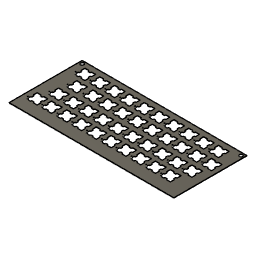
Metal_dome_array_layer_0.4mm (Autodesk Fusion 360 design; units mm, degrees)
Autodesk Fusion 360 part; units mm, degrees
(part 1 of 4)
sketch "스케치1" plane through (0, 0, 0) normal (0, 0, 1) x (1, 0, 0)
  line L0 (0, 69) -> (155.5, 69)
  line L1 (155.5, 69) -> (155.5, 0)
  line L2 (155.5, 0) -> (0, 0)
  line L3 (0, 0) -> (0, 69)
  line L4 (12.673, 10.08) -> (26.673, 10.08) construction
  line L5 (26.673, 10.08) -> (40.673, 10.08) construction
  line L6 (40.673, 10.08) -> (54.673, 10.08) construction
  line L7 (54.673, 10.08) -> (68.673, 10.08) construction
  line L8 (68.673, 10.08) -> (82.673, 10.08) construction
  line L9 (82.673, 10.08) -> (96.673, 10.08) construction
  line L10 (96.673, 10.08) -> (110.673, 10.08) construction
  line L11 (110.673, 10.08) -> (124.673, 10.08) construction
  line L12 (124.673, 10.08) -> (138.673, 10.08) construction
  circle A0 centre (12.673, 10.08) radius 5.05
  circle A1 centre (26.673, 10.08) radius 5.05
  circle A2 centre (40.673, 10.08) radius 5.05
  circle A3 centre (54.673, 10.08) radius 5.05
  circle A4 centre (68.673, 10.08) radius 5.05
  circle A5 centre (82.673, 10.08) radius 5.05
  circle A6 centre (96.673, 10.08) radius 5.05
  circle A7 centre (110.673, 10.08) radius 5.05
  circle A8 centre (124.673, 10.08) radius 5.05
  circle A9 centre (138.673, 10.08) radius 5.05
  line L13 (19.024, 24.05) -> (34.274, 24.05) construction
  line L14 (34.274, 24.05) -> (48.244, 24.05) construction
  line L15 (48.244, 24.05) -> (62.214, 24.05) construction
  line L16 (62.214, 24.05) -> (76.184, 24.05) construction
  line L17 (76.184, 24.05) -> (90.154, 24.05) construction
  line L18 (90.154, 24.05) -> (104.124, 24.05) construction
  line L19 (104.124, 24.05) -> (118.094, 24.05) construction
  line L20 (118.094, 24.05) -> (132.064, 24.05) construction
  line L21 (132.064, 24.05) -> (146.034, 24.05) construction
  circle A10 centre (19.024, 24.05) radius 5.05
  circle A11 centre (34.274, 24.05) radius 5.05
  circle A12 centre (48.244, 24.05) radius 5.05
  circle A13 centre (62.214, 24.05) radius 5.05
  circle A14 centre (76.184, 24.05) radius 5.05
  circle A15 centre (90.154, 24.05) radius 5.05
  circle A16 centre (104.124, 24.05) radius 5.05
  circle A17 centre (118.094, 24.05) radius 5.05
  circle A18 centre (132.064, 24.05) radius 5.05
  circle A19 centre (146.034, 24.05) radius 5.05
  line L22 (16.483, 38.655) -> (30.453, 38.655) construction
  line L23 (30.453, 38.655) -> (44.423, 38.655) construction
  line L24 (44.423, 38.655) -> (58.393, 38.655) construction
  line L25 (58.393, 38.655) -> (72.363, 38.655) construction
  circle A20 centre (16.483, 38.655) radius 5.05
  circle A21 centre (30.453, 38.655) radius 5.05
  circle A22 centre (44.423, 38.655) radius 5.05
  circle A23 centre (58.393, 38.655) radius 5.05
  circle A24 centre (72.363, 38.655) radius 5.05
  circle A25 centre (86.333, 38.655) radius 5.05
  circle A26 centre (100.303, 38.655) radius 5.05
  circle A27 centre (114.273, 38.655) radius 5.05
  circle A28 centre (128.243, 38.655) radius 5.05
  circle A29 centre (142.213, 38.655) radius 5.05
  line L26 (72.363, 38.655) -> (86.333, 38.655) construction
  line L27 (86.333, 38.655) -> (100.303, 38.655) construction
  line L28 (100.303, 38.655) -> (114.273, 38.655) construction
  line L29 (114.273, 38.655) -> (128.243, 38.655) construction
  line L30 (128.243, 38.655) -> (142.213, 38.655) construction
  line L31 (10.13, 52.625) -> (23.78, 52.625) construction
  line L32 (23.78, 52.625) -> (38.07, 52.625) construction
  line L33 (38.07, 52.625) -> (52.04, 52.625) construction
  line L34 (52.04, 52.625) -> (66.01, 52.625) construction
  line L35 (66.01, 52.625) -> (79.98, 52.625) construction
  line L36 (79.98, 52.625) -> (93.95, 52.625) construction
  line L37 (93.95, 52.625) -> (107.92, 52.625) construction
  line L38 (107.92, 52.625) -> (121.89, 52.625) construction
  line L39 (121.89, 52.625) -> (135.86, 52.625) construction
  circle A30 centre (10.13, 52.625) radius 5.05
  circle A31 centre (23.78, 52.625) radius 5.05
  circle A32 centre (38.07, 52.625) radius 5.05
  circle A33 centre (52.04, 52.625) radius 5.05
  circle A34 centre (79.98, 52.625) radius 5.05
  circle A35 centre (93.95, 52.625) radius 5.05
  circle A36 centre (107.92, 52.625) radius 5.05
  circle A37 centre (121.89, 52.625) radius 5.05
  circle A38 centre (135.86, 52.625) radius 5.05
  circle A39 centre (66.01, 52.625) radius 5.05
  circle A40 centre (2.8, 2.8) radius 1.55
  circle A41 centre (152.7, 2.8) radius 1.55
  circle A42 centre (3.81, 65.25) radius 0.95
  circle A43 centre (151.69, 65.25) radius 0.95
  line L40 (0.4, 68.6) -> (155.1, 68.6)
  line L41 (155.1, 68.6) -> (155.1, 0.4)
  line L42 (155.1, 0.4) -> (0.4, 0.4)
  line L43 (0.4, 0.4) -> (0.4, 68.6)
  dimension "d1" = 155.5
  dimension "d2" = 69
  dimension "d3" = 14
  dimension "d4" = 12.673
  dimension "d5" = 10.08
  dimension "d6" = 10.1
  dimension "d8" = 15.25
  dimension "d9" = 13.97
  dimension "d10" = 19.024
  dimension "d11" = 13.97
  dimension "d12" = 13.97
  dimension "d13" = 14.605
  dimension "d14" = 16.483
  dimension "d15" = 13.65
  dimension "d16" = 14.29
  dimension "d17" = 13.97
  dimension "d18" = 10.13
  dimension "d19" = 13.97
  dimension "d20" = 3.1
  dimension "d21" = 2.8
  dimension "d22" = 2.8
  dimension "d23" = 2.8
  dimension "d24" = 2.8
  dimension "d25" = 3.81
  dimension "d26" = 65.25
  dimension "d27" = 1.9
  dimension "d28" = 3.81
  dimension "d29" = 65.25
  dimension "d45" = 0.4
  constraint horizontal L0
  constraint vertical L1
  constraint horizontal L2
  constraint vertical L3
  constraint coincident L2.end L3.start
  constraint horizontal L4
  constraint parallel L4 L5
  constraint parallel L5 L6
  constraint parallel L6 L7
  constraint parallel L6 L8
  constraint parallel L8 L9
  constraint parallel L8 L10
  constraint parallel L10 L11
  constraint parallel L10 L12
  constraint equal L4 L5
  constraint equal L4 L6
  constraint equal L4 L7
  constraint equal L4 L8
  constraint equal L4 L9
  constraint equal L4 L10
  constraint equal L4 L11
  constraint equal L4 L12
  constraint coincident L4.start A0.centre
  constraint coincident L4.end L5.start
  constraint coincident L5.end L6.start
  constraint coincident L6.end L7.start
  constraint coincident L7.end L8.start
  constraint coincident L8.end L9.start
  constraint coincident L9.end L10.start
  constraint coincident L10.end L11.start
  constraint coincident L11.end L12.start
  constraint coincident L12.end A9.centre
  constraint equal A0 A1
  constraint equal A0 A2
  constraint equal A0 A3
  constraint equal A0 A4
  constraint equal A0 A5
  constraint equal A0 A6
  constraint equal A0 A7
  constraint equal A0 A8
  constraint equal A0 A9
  constraint parallel L0 L13
  constraint parallel L0 L14
  constraint parallel L0 L15
  constraint parallel L15 L16
  constraint parallel L16 L17
  constraint parallel L16 L18
  constraint parallel L18 L19
  constraint parallel L18 L20
  constraint parallel L18 L21
  constraint equal L15 L16
  constraint equal L15 L17
  constraint equal L15 L18
  constraint equal L15 L19
  constraint equal L15 L20
  constraint equal L15 L21
  constraint equal L14 L15
  constraint coincident L21.end A19.centre
  constraint coincident L20.end L21.start
  constraint coincident L19.end L20.start
  constraint coincident L18.end L19.start
  constraint coincident L17.end L18.start
  constraint coincident L16.end L17.start
  constraint coincident L15.end L16.start
  constraint coincident L14.end L15.start
  constraint coincident L13.end L14.start
  constraint coincident L13.start A10.centre
  constraint equal A0 A10
  constraint equal A0 A11
  constraint equal A0 A12
  constraint equal A0 A13
  constraint equal A0 A14
  constraint equal A0 A15
  constraint equal A0 A16
  constraint equal A0 A17
  constraint equal A0 A18
  constraint equal A0 A19
  constraint horizontal L22
  constraint parallel L22 L23
  constraint parallel L23 L24
  constraint parallel L24 L25
  constraint equal L22 L23
  constraint equal L22 L24
  constraint equal L22 L25
  constraint coincident L22.start A20.centre
  constraint coincident L22.end L23.start
  constraint coincident L23.end L24.start
  constraint coincident L24.end L25.start
  constraint coincident L25.end A24.centre
  constraint parallel L25 L26
  constraint parallel L25 L27
  constraint parallel L25 L28
  constraint parallel L25 L29
  constraint parallel L25 L30
  constraint equal L22 L26
  constraint equal L22 L27
  constraint equal L22 L28
  constraint equal L22 L29
  constraint coincident A25.centre L26.end
  constraint coincident A26.centre L27.end
  constraint coincident A27.centre L28.end
  constraint coincident A28.centre L29.end
  constraint coincident A29.centre L30.end
  constraint equal L22 L30
  constraint equal A0 A20
  constraint equal A0 A21
  constraint equal A0 A22
  constraint equal A0 A23
  constraint equal A0 A24
  constraint equal A0 A25
  constraint equal A0 A26
  constraint equal A0 A27
  constraint equal A0 A28
  constraint equal A0 A29
  constraint horizontal L31
  constraint parallel L31 L32
  constraint parallel L32 L33
  constraint parallel L33 L34
  constraint parallel L33 L35
  constraint parallel L35 L36
  constraint parallel L36 L37
  constraint parallel L37 L38
  constraint parallel L38 L39
  constraint equal L33 L34
  constraint equal L33 L35
  constraint equal L33 L36
  constraint equal L33 L37
  constraint equal L33 L38
  constraint equal L33 L39
  constraint coincident L31.start A30.centre
  constraint coincident L31.end L32.start
  constraint coincident L32.end L33.start
  constraint coincident L33.end L34.start
  constraint coincident L34.end L35.start
  constraint coincident L35.end L36.start
  constraint coincident L36.end L37.start
  constraint coincident L37.end L38.start
  constraint coincident L38.end L39.start
  constraint coincident L39.end A38.centre
  constraint equal A0 A30
  constraint equal A0 A31
  constraint equal A0 A32
  constraint equal A0 A33
  constraint equal A0 A39
  constraint equal A0 A34
  constraint equal A0 A35
  constraint equal A0 A36
  constraint equal A0 A37
  constraint equal A0 A38
  constraint equal A40 A41
  constraint equal A42 A43
  measures "d1" distance of L1.end L2.end
  measures "d2" distance of L0.start L2.end
  measures "d3" distance of L4.start L4.end
  measures "d4" distance of L3 L4.start
  measures "d5" distance of L2 L4.start
  measures "d6" diameter of A0
  measures "d8" distance of L13.start L13.end
  measures "d9" distance of L13.end L14.end
  measures "d10" distance of L3 L13.start
  measures "d11" distance of L4 L13.start
  measures "d12" distance of L22.start L22.end
  measures "d13" distance of L13 L22.start
  measures "d14" distance of L3 L22.start
  measures "d15" distance of L31.start L31.end
  measures "d16" distance of L31.end L32.end
  measures "d17" distance of L32.end L33.end
  measures "d18" distance of L3 L31.start
  measures "d19" distance of L22 L31.start
  measures "d20" diameter of A40
  measures "d21" distance of L2 A40.centre
  measures "d22" distance of L3 A40.centre
  measures "d23" distance of L2 A41.centre
  measures "d24" distance of L1 A41.centre
  measures "d25" distance of L3 A42.centre
  measures "d26" distance of L2 A42.centre
  measures "d27" diameter of A42
  measures "d28" distance of L1 A43.centre
  measures "d29" distance of L2 A43.centre
sketch "스케치2" plane through (0, 0, 0) normal (0, 0, 1) x (1, 0, 0)
  line L0 (5.08, 57.675) -> (15.18, 57.675)
  line L1 (15.18, 57.675) -> (15.18, 47.575)
  line L2 (15.18, 47.575) -> (5.08, 47.575)
  line L3 (5.08, 47.575) -> (5.08, 57.675)
  line L4 (18.73, 57.675) -> (28.83, 57.675)
  line L5 (28.83, 57.675) -> (28.83, 47.575)
  line L6 (28.83, 47.575) -> (18.73, 47.575)
  line L7 (18.73, 47.575) -> (18.73, 57.675)
  line L8 (33.02, 57.675) -> (43.12, 57.675)
  line L9 (43.12, 57.675) -> (43.12, 47.575)
  line L10 (43.12, 47.575) -> (33.02, 47.575)
  line L11 (33.02, 47.575) -> (33.02, 57.675)
  line L12 (46.99, 57.675) -> (57.09, 57.675)
  line L13 (57.09, 57.675) -> (57.09, 47.575)
  line L14 (57.09, 47.575) -> (46.99, 47.575)
  line L15 (46.99, 47.575) -> (46.99, 57.675)
  line L16 (60.96, 57.675) -> (71.06, 57.675)
  line L17 (71.06, 57.675) -> (71.06, 47.575)
  line L18 (71.06, 47.575) -> (60.96, 47.575)
  line L19 (60.96, 47.575) -> (60.96, 57.675)
  line L20 (74.93, 57.675) -> (85.03, 57.675)
  line L21 (85.03, 57.675) -> (85.03, 47.575)
  line L22 (85.03, 47.575) -> (74.93, 47.575)
  line L23 (74.93, 47.575) -> (74.93, 57.675)
  line L24 (88.9, 57.675) -> (99, 57.675)
  line L25 (99, 57.675) -> (99, 47.575)
  line L26 (99, 47.575) -> (88.9, 47.575)
  line L27 (88.9, 47.575) -> (88.9, 57.675)
  line L28 (102.87, 57.675) -> (112.97, 57.675)
  line L29 (112.97, 57.675) -> (112.97, 47.575)
  line L30 (112.97, 47.575) -> (102.87, 47.575)
  line L31 (102.87, 47.575) -> (102.87, 57.675)
  line L32 (116.84, 57.675) -> (126.94, 57.675)
  line L33 (126.94, 57.675) -> (126.94, 47.575)
  line L34 (126.94, 47.575) -> (116.84, 47.575)
  line L35 (116.84, 47.575) -> (116.84, 57.675)
  line L36 (130.81, 57.675) -> (140.91, 57.675)
  line L37 (140.91, 57.675) -> (140.91, 47.575)
  line L38 (140.91, 47.575) -> (130.81, 47.575)
  line L39 (130.81, 47.575) -> (130.81, 57.675)
  line L40 (11.433, 43.705) -> (21.533, 43.705)
  line L41 (21.533, 43.705) -> (21.533, 33.605)
  line L42 (21.533, 33.605) -> (11.433, 33.605)
  line L43 (11.433, 33.605) -> (11.433, 43.705)
  line L44 (25.403, 43.705) -> (35.503, 43.705)
  line L45 (35.503, 43.705) -> (35.503, 33.605)
  line L46 (35.503, 33.605) -> (25.403, 33.605)
  line L47 (25.403, 33.605) -> (25.403, 43.705)
  line L48 (39.373, 43.705) -> (49.473, 43.705)
  line L49 (49.473, 43.705) -> (49.473, 33.605)
  line L50 (49.473, 33.605) -> (39.373, 33.605)
  line L51 (39.373, 33.605) -> (39.373, 43.705)
  line L52 (53.343, 43.705) -> (63.443, 43.705)
  line L53 (63.443, 43.705) -> (63.443, 33.605)
  line L54 (63.443, 33.605) -> (53.343, 33.605)
  line L55 (53.343, 33.605) -> (53.343, 43.705)
  line L56 (67.313, 43.705) -> (77.413, 43.705)
  line L57 (77.413, 43.705) -> (77.413, 33.605)
  line L58 (77.413, 33.605) -> (67.313, 33.605)
  line L59 (67.313, 33.605) -> (67.313, 43.705)
  line L60 (81.283, 43.705) -> (91.383, 43.705)
  line L61 (91.383, 43.705) -> (91.383, 33.605)
  line L62 (91.383, 33.605) -> (81.283, 33.605)
  line L63 (81.283, 33.605) -> (81.283, 43.705)
  line L64 (95.253, 43.705) -> (105.353, 43.705)
  line L65 (105.353, 43.705) -> (105.353, 33.605)
  line L66 (105.353, 33.605) -> (95.253, 33.605)
  line L67 (95.253, 33.605) -> (95.253, 43.705)
  line L68 (109.223, 43.705) -> (119.323, 43.705)
  line L69 (119.323, 43.705) -> (119.323, 33.605)
  line L70 (119.323, 33.605) -> (109.223, 33.605)
  line L71 (109.223, 33.605) -> (109.223, 43.705)
  line L72 (123.193, 43.705) -> (133.293, 43.705)
  line L73 (133.293, 43.705) -> (133.293, 33.605)
  line L74 (133.293, 33.605) -> (123.193, 33.605)
  line L75 (123.193, 33.605) -> (123.193, 43.705)
  line L76 (137.163, 43.705) -> (147.263, 43.705)
  line L77 (147.263, 43.705) -> (147.263, 33.605)
  line L78 (147.263, 33.605) -> (137.163, 33.605)
  line L79 (137.163, 33.605) -> (137.163, 43.705)
  line L80 (140.984, 29.1) -> (151.084, 29.1)
  line L81 (151.084, 29.1) -> (151.084, 19)
  line L82 (151.084, 19) -> (140.984, 19)
  line L83 (140.984, 19) -> (140.984, 29.1)
  line L84 (127.014, 29.1) -> (137.114, 29.1)
  line L85 (137.114, 29.1) -> (137.114, 19)
  line L86 (137.114, 19) -> (127.014, 19)
  line L87 (127.014, 19) -> (127.014, 29.1)
  line L88 (113.044, 29.1) -> (123.144, 29.1)
  line L89 (123.144, 29.1) -> (123.144, 19)
  line L90 (123.144, 19) -> (113.044, 19)
  line L91 (113.044, 19) -> (113.044, 29.1)
  line L92 (99.074, 29.1) -> (109.174, 29.1)
  line L93 (109.174, 29.1) -> (109.174, 19)
  line L94 (109.174, 19) -> (99.074, 19)
  line L95 (99.074, 19) -> (99.074, 29.1)
  line L96 (85.104, 29.1) -> (95.204, 29.1)
  line L97 (95.204, 29.1) -> (95.204, 19)
  line L98 (95.204, 19) -> (85.104, 19)
  line L99 (85.104, 19) -> (85.104, 29.1)
  line L100 (71.134, 29.1) -> (81.234, 29.1)
  line L101 (81.234, 29.1) -> (81.234, 19)
  line L102 (81.234, 19) -> (71.134, 19)
  line L103 (71.134, 19) -> (71.134, 29.1)
  line L104 (57.164, 29.1) -> (67.264, 29.1)
  line L105 (67.264, 29.1) -> (67.264, 19)
  line L106 (67.264, 19) -> (57.164, 19)
  line L107 (57.164, 19) -> (57.164, 29.1)
  line L108 (43.194, 29.1) -> (53.294, 29.1)
  line L109 (53.294, 29.1) -> (53.294, 19)
  line L110 (53.294, 19) -> (43.194, 19)
  line L111 (43.194, 19) -> (43.194, 29.1)
  line L112 (29.224, 29.1) -> (39.324, 29.1)
  line L113 (39.324, 29.1) -> (39.324, 19)
  line L114 (39.324, 19) -> (29.224, 19)
  line L115 (29.224, 19) -> (29.224, 29.1)
  line L116 (13.974, 29.1) -> (24.074, 29.1)
  line L117 (24.074, 29.1) -> (24.074, 19)
  line L118 (24.074, 19) -> (13.974, 19)
  line L119 (13.974, 19) -> (13.974, 29.1)
  line L120 (7.623, 15.13) -> (17.723, 15.13)
  line L121 (17.723, 15.13) -> (17.723, 5.03)
  line L122 (17.723, 5.03) -> (7.623, 5.03)
  line L123 (7.623, 5.03) -> (7.623, 15.13)
  line L124 (21.623, 15.13) -> (31.723, 15.13)
  line L125 (31.723, 15.13) -> (31.723, 5.03)
  line L126 (31.723, 5.03) -> (21.623, 5.03)
  line L127 (21.623, 5.03) -> (21.623, 15.13)
  line L128 (35.623, 15.13) -> (45.723, 15.13)
  line L129 (45.723, 15.13) -> (45.723, 5.03)
  line L130 (45.723, 5.03) -> (35.623, 5.03)
  line L131 (35.623, 5.03) -> (35.623, 15.13)
  line L132 (49.623, 15.13) -> (59.723, 15.13)
  line L133 (59.723, 15.13) -> (59.723, 5.03)
  line L134 (59.723, 5.03) -> (49.623, 5.03)
  line L135 (49.623, 5.03) -> (49.623, 15.13)
  line L136 (63.623, 15.13) -> (73.723, 15.13)
  line L137 (73.723, 15.13) -> (73.723, 5.03)
  line L138 (73.723, 5.03) -> (63.623, 5.03)
  line L139 (63.623, 5.03) -> (63.623, 15.13)
  line L140 (77.623, 15.13) -> (87.723, 15.13)
  line L141 (87.723, 15.13) -> (87.723, 5.03)
  line L142 (87.723, 5.03) -> (77.623, 5.03)
  line L143 (77.623, 5.03) -> (77.623, 15.13)
  line L144 (91.623, 15.13) -> (101.723, 15.13)
  line L145 (101.723, 15.13) -> (101.723, 5.03)
  line L146 (101.723, 5.03) -> (91.623, 5.03)
  line L147 (91.623, 5.03) -> (91.623, 15.13)
  line L148 (105.623, 15.13) -> (115.723, 15.13)
  line L149 (115.723, 15.13) -> (115.723, 5.03)
  line L150 (115.723, 5.03) -> (105.623, 5.03)
  line L151 (105.623, 5.03) -> (105.623, 15.13)
  line L152 (119.623, 15.13) -> (129.723, 15.13)
  line L153 (129.723, 15.13) -> (129.723, 5.03)
  line L154 (129.723, 5.03) -> (119.623, 5.03)
  line L155 (119.623, 5.03) -> (119.623, 15.13)
  line L156 (133.623, 15.13) -> (143.723, 15.13)
  line L157 (143.723, 15.13) -> (143.723, 5.03)
  line L158 (143.723, 5.03) -> (133.623, 5.03)
  line L159 (133.623, 5.03) -> (133.623, 15.13)
  circle A0 centre (10.13, 52.625) radius 5.05
  circle A1 centre (23.78, 52.625) radius 5.05
  circle A2 centre (38.07, 52.625) radius 5.05
  circle A3 centre (52.04, 52.625) radius 5.05
  circle A4 centre (66.01, 52.625) radius 5.05
  circle A5 centre (79.98, 52.625) radius 5.05
  circle A6 centre (93.95, 52.625) radius 5.05
  circle A7 centre (107.92, 52.625) radius 5.05
  circle A8 centre (121.89, 52.625) radius 5.05
  circle A9 centre (135.86, 52.625) radius 5.05
  circle A10 centre (16.483, 38.655) radius 5.05
  circle A11 centre (30.453, 38.655) radius 5.05
  circle A12 centre (44.423, 38.655) radius 5.05
  circle A13 centre (58.393, 38.655) radius 5.05
  circle A14 centre (72.363, 38.655) radius 5.05
  circle A15 centre (86.333, 38.655) radius 5.05
  circle A16 centre (100.303, 38.655) radius 5.05
  circle A17 centre (114.273, 38.655) radius 5.05
  circle A18 centre (128.243, 38.655) radius 5.05
  circle A19 centre (142.213, 38.655) radius 5.05
  circle A20 centre (19.024, 24.05) radius 5.05
  circle A21 centre (34.274, 24.05) radius 5.05
  circle A22 centre (48.244, 24.05) radius 5.05
  circle A23 centre (76.184, 24.05) radius 5.05
  circle A24 centre (62.214, 24.05) radius 5.05
  circle A25 centre (90.154, 24.05) radius 5.05
  circle A26 centre (104.124, 24.05) radius 5.05
  circle A27 centre (118.094, 24.05) radius 5.05
  circle A28 centre (132.064, 24.05) radius 5.05
  circle A29 centre (146.034, 24.05) radius 5.05
  circle A30 centre (12.673, 10.08) radius 5.05
  circle A31 centre (26.673, 10.08) radius 5.05
  circle A32 centre (40.673, 10.08) radius 5.05
  circle A33 centre (54.673, 10.08) radius 5.05
  circle A34 centre (68.673, 10.08) radius 5.05
  circle A35 centre (82.673, 10.08) radius 5.05
  circle A36 centre (96.673, 10.08) radius 5.05
  circle A37 centre (110.673, 10.08) radius 5.05
  circle A38 centre (124.673, 10.08) radius 5.05
  circle A39 centre (138.673, 10.08) radius 5.05
  line L160 (5.08, 55.7658) -> (6.9892, 57.675)
  line L161 (6.0346, 56.7204) -> (5.08, 57.675) construction
  line L162 (137.163, 41.7958) -> (139.0722, 43.705)
  line L163 (137.163, 43.705) -> (137.3462, 43.705) construction
  line L164 (137.163, 43.705) -> (138.1176, 42.7504) construction
  line L165 (13.974, 27.1908) -> (15.8832, 29.1)
  line L166 (13.974, 29.1) -> (14.9286, 28.1454) construction
  line L167 (133.623, 13.2208) -> (135.5322, 15.13)
  line L168 (133.623, 15.13) -> (134.5776, 14.1754) construction
  circle A40 centre (5.7164, 57.0386) radius 0.45
  circle A41 centre (14.6104, 28.4636) radius 0.45
  circle A42 centre (137.7994, 43.0686) radius 0.45
  circle A43 centre (134.2594, 14.4936) radius 0.45
  line L169 (25.403, 41.7958) -> (27.3122, 43.705)
  line L170 (53.343, 41.7958) -> (55.2522, 43.705)
  line L171 (81.283, 41.7958) -> (83.1922, 43.705)
  line L172 (109.223, 41.7958) -> (111.1322, 43.705)
  line L173 (43.194, 27.1908) -> (45.1032, 29.1)
  line L174 (18.73, 55.7658) -> (20.6392, 57.675)
  line L175 (33.02, 55.7658) -> (34.9292, 57.675)
  line L176 (46.99, 55.7658) -> (48.8992, 57.675)
  line L177 (60.96, 55.7658) -> (62.8692, 57.675)
  line L178 (74.93, 55.7658) -> (76.8392, 57.675)
  line L179 (88.9, 55.7658) -> (90.8092, 57.675)
  line L180 (102.87, 55.7658) -> (104.7792, 57.675)
  line L181 (116.84, 55.7658) -> (118.7492, 57.675)
  line L182 (130.81, 55.7658) -> (132.7192, 57.675)
  line L183 (18.73, 57.675) -> (19.6846, 56.7204) construction
  line L184 (33.02, 57.675) -> (33.9746, 56.7204) construction
  line L185 (46.99, 57.675) -> (47.9446, 56.7204) construction
  line L186 (60.96, 57.675) -> (61.9146, 56.7204) construction
  line L187 (74.93, 57.675) -> (75.8846, 56.7204) construction
  line L188 (88.9, 57.675) -> (89.8546, 56.7204) construction
  line L189 (102.87, 57.675) -> (103.8246, 56.7204) construction
  line L190 (116.84, 57.675) -> (117.7946, 56.7204) construction
  line L191 (130.81, 57.675) -> (131.7646, 56.7204) construction
  circle A44 centre (19.3664, 57.0386) radius 0.45
  circle A45 centre (33.6564, 57.0386) radius 0.45
  circle A46 centre (47.6264, 57.0386) radius 0.45
  circle A47 centre (61.5964, 57.0386) radius 0.45
  circle A48 centre (75.5664, 57.0386) radius 0.45
  circle A49 centre (89.5364, 57.0386) radius 0.45
  circle A50 centre (103.5064, 57.0386) radius 0.45
  circle A51 centre (117.4764, 57.0386) radius 0.45
  circle A52 centre (131.4464, 57.0386) radius 0.45
  line L192 (11.433, 41.7958) -> (13.3422, 43.705)
  line L193 (39.373, 41.7958) -> (41.2822, 43.705)
  line L194 (67.313, 41.7958) -> (69.2222, 43.705)
  line L195 (95.253, 41.7958) -> (97.1622, 43.705)
  line L196 (123.193, 41.7958) -> (125.1022, 43.705)
  line L197 (11.433, 43.705) -> (12.3876, 42.7504) construction
  line L198 (25.403, 43.705) -> (26.3576, 42.7504) construction
  line L199 (39.373, 43.705) -> (40.3276, 42.7504) construction
  line L200 (53.343, 43.705) -> (54.2976, 42.7504) construction
  line L201 (67.313, 43.705) -> (68.2676, 42.7504) construction
  line L202 (81.283, 43.705) -> (82.2376, 42.7504) construction
  line L203 (95.253, 43.705) -> (96.2076, 42.7504) construction
  line L204 (109.223, 43.705) -> (110.1776, 42.7504) construction
  line L205 (123.193, 43.705) -> (124.1476, 42.7504) construction
  circle A53 centre (12.0694, 43.0686) radius 0.45
  circle A54 centre (26.0394, 43.0686) radius 0.45
  circle A55 centre (40.0094, 43.0686) radius 0.45
  circle A56 centre (53.9794, 43.0686) radius 0.45
  circle A57 centre (67.9494, 43.0686) radius 0.45
  circle A58 centre (81.9194, 43.0686) radius 0.45
  circle A59 centre (95.8894, 43.0686) radius 0.45
  circle A60 centre (109.8594, 43.0686) radius 0.45
  circle A61 centre (123.8294, 43.0686) radius 0.45
  line L206 (29.224, 27.1908) -> (31.1332, 29.1)
  line L207 (57.164, 27.1908) -> (59.0732, 29.1)
  line L208 (71.134, 27.1908) -> (73.0432, 29.1)
  line L209 (85.104, 27.1908) -> (87.0132, 29.1)
  line L210 (99.074, 27.1908) -> (100.9832, 29.1)
  line L211 (113.044, 27.1908) -> (114.9532, 29.1)
  line L212 (127.014, 27.1908) -> (128.9232, 29.1)
  line L213 (140.984, 27.1908) -> (142.8932, 29.1)
  line L214 (127.014, 29.1) -> (127.9686, 28.1454) construction
  line L215 (113.044, 29.1) -> (113.9986, 28.1454) construction
  line L216 (99.074, 29.1) -> (100.0286, 28.1454) construction
  line L217 (85.104, 29.1) -> (86.0586, 28.1454) construction
  line L218 (71.134, 29.1) -> (72.0886, 28.1454) construction
  line L219 (57.164, 29.1) -> (58.1186, 28.1454) construction
  line L220 (43.194, 29.1) -> (44.1486, 28.1454) construction
  line L221 (29.224, 29.1) -> (30.1786, 28.1454) construction
  line L222 (140.984, 29.1) -> (141.9386, 28.1454) construction
  circle A62 centre (29.8604, 28.4636) radius 0.45
  circle A63 centre (57.8004, 28.4636) radius 0.45
  circle A64 centre (43.8304, 28.4636) radius 0.45
  circle A65 centre (85.7404, 28.4636) radius 0.45
  circle A66 centre (71.7704, 28.4636) radius 0.45
  circle A67 centre (113.6804, 28.4636) radius 0.45
  circle A68 centre (99.7104, 28.4636) radius 0.45
  circle A69 centre (141.6204, 28.4636) radius 0.45
  circle A70 centre (127.6504, 28.4636) radius 0.45
  line L223 (119.623, 13.2208) -> (121.5322, 15.13)
  line L224 (105.623, 13.2208) -> (107.5322, 15.13)
  line L225 (91.623, 13.2208) -> (93.5322, 15.13)
  line L226 (77.623, 13.2208) -> (79.5322, 15.13)
  line L227 (63.623, 13.2208) -> (65.5322, 15.13)
  line L228 (49.623, 13.2208) -> (51.5322, 15.13)
  line L229 (35.623, 13.2208) -> (37.5322, 15.13)
  line L230 (21.623, 13.2208) -> (23.5322, 15.13)
  line L231 (7.623, 13.2208) -> (9.5322, 15.13)
  line L232 (119.623, 15.13) -> (120.5776, 14.1754) construction
  line L233 (105.623, 15.13) -> (106.5776, 14.1754) construction
  line L234 (91.623, 15.13) -> (92.5776, 14.1754) construction
  line L235 (77.623, 15.13) -> (78.5776, 14.1754) construction
  line L236 (63.623, 15.13) -> (64.5776, 14.1754) construction
  line L237 (49.623, 15.13) -> (50.5776, 14.1754) construction
  line L238 (35.623, 15.13) -> (36.5776, 14.1754) construction
  line L239 (21.623, 15.13) -> (22.5776, 14.1754) construction
  line L240 (7.623, 15.13) -> (8.5776, 14.1754) construction
  circle A71 centre (120.2594, 14.4936) radius 0.45
  circle A72 centre (106.2594, 14.4936) radius 0.45
  circle A73 centre (92.2594, 14.4936) radius 0.45
  circle A74 centre (78.2594, 14.4936) radius 0.45
  circle A75 centre (64.2594, 14.4936) radius 0.45
  circle A76 centre (50.2594, 14.4936) radius 0.45
  circle A77 centre (36.2594, 14.4936) radius 0.45
  circle A78 centre (22.2594, 14.4936) radius 0.45
  circle A79 centre (8.2594, 14.4936) radius 0.45
  dimension "d51" = 45
  dimension "d52" = 1.35
  dimension "d53" = 45
  dimension "d55" = 45
  dimension "d56" = 45
  dimension "d61" = 0.9
  dimension "d63" = 45
  dimension "d64" = 45
  dimension "d65" = 45
  dimension "d66" = 45
  dimension "d67" = 45
  dimension "d68" = 45
  dimension "d69" = 45
  dimension "d70" = 45
  dimension "d72" = 45
  dimension "d74" = 45
  dimension "d75" = 45
  dimension "d76" = 45
  dimension "d77" = 45
  dimension "d78" = 45
  dimension "d80" = 45
  dimension "d81" = 45
  dimension "d82" = 45
  dimension "d83" = 45
  dimension "d84" = 45
  dimension "d85" = 45
  dimension "d86" = 45
  dimension "d87" = 45
  dimension "d88" = 45
  dimension "d89" = 45
  dimension "d91" = 45
  dimension "d92" = 45
  dimension "d93" = 45
  dimension "d94" = 45
  dimension "d95" = 45
  dimension "d96" = 45
  dimension "d97" = 45
  dimension "d98" = 45
  dimension "d99" = 45
  dimension "d100" = 45
  dimension "d101" = 45
  dimension "d102" = 45
  constraint horizontal L0
  constraint vertical L1
  constraint horizontal L2
  constraint vertical L3
  constraint horizontal L4
  constraint vertical L5
  constraint horizontal L6
  constraint vertical L7
  constraint horizontal L8
  constraint vertical L9
  constraint horizontal L10
  constraint vertical L11
  constraint horizontal L12
  constraint vertical L13
  constraint horizontal L14
  constraint vertical L15
  constraint horizontal L16
  constraint vertical L17
  constraint horizontal L18
  constraint vertical L19
  constraint horizontal L20
  constraint vertical L21
  constraint horizontal L22
  constraint vertical L23
  constraint horizontal L24
  constraint vertical L25
  constraint horizontal L26
  constraint vertical L27
  constraint horizontal L28
  constraint vertical L29
  constraint horizontal L30
  constraint vertical L31
  constraint horizontal L32
  constraint vertical L33
  constraint horizontal L34
  constraint vertical L35
  constraint horizontal L36
  constraint vertical L37
  constraint horizontal L38
  constraint vertical L39
  constraint horizontal L40
  constraint vertical L41
  constraint horizontal L42
  constraint vertical L43
  constraint horizontal L44
  constraint vertical L45
  constraint horizontal L46
  constraint vertical L47
  constraint horizontal L48
  constraint vertical L49
  constraint horizontal L50
  constraint vertical L51
  constraint horizontal L52
  constraint vertical L53
  constraint horizontal L54
  constraint vertical L55
  constraint horizontal L56
  constraint vertical L57
  constraint horizontal L58
  constraint vertical L59
  constraint horizontal L60
  constraint vertical L61
  constraint horizontal L62
  constraint vertical L63
  constraint horizontal L64
  constraint vertical L65
  constraint horizontal L66
  constraint vertical L67
  constraint horizontal L68
  constraint vertical L69
  constraint horizontal L70
  constraint vertical L71
  constraint horizontal L72
  constraint vertical L73
  constraint horizontal L74
  constraint vertical L75
  constraint horizontal L76
  constraint vertical L77
  constraint horizontal L78
  constraint vertical L79
  constraint horizontal L80
  constraint vertical L81
  constraint horizontal L82
  constraint vertical L83
  constraint horizontal L84
  constraint vertical L85
  constraint horizontal L86
  constraint vertical L87
  constraint horizontal L88
  constraint vertical L89
  constraint horizontal L90
  constraint vertical L91
  constraint horizontal L92
  constraint vertical L93
  constraint horizontal L94
  constraint vertical L95
  constraint horizontal L96
  constraint vertical L97
  constraint horizontal L98
  constraint vertical L99
  constraint horizontal L100
  constraint vertical L101
  constraint horizontal L102
  constraint vertical L103
  constraint horizontal L104
  constraint vertical L105
  constraint horizontal L106
  constraint vertical L107
  constraint horizontal L108
  constraint vertical L109
  constraint horizontal L110
  constraint vertical L111
  constraint horizontal L112
  constraint vertical L113
  constraint horizontal L114
  constraint vertical L115
  constraint horizontal L116
  constraint vertical L117
  constraint horizontal L118
  constraint vertical L119
  constraint horizontal L120
  constraint vertical L121
  constraint horizontal L122
  constraint vertical L123
  constraint horizontal L124
  constraint vertical L125
  constraint horizontal L126
  constraint vertical L127
  constraint horizontal L128
  constraint vertical L129
  constraint horizontal L130
  constraint vertical L131
  constraint horizontal L132
  constraint vertical L133
  constraint horizontal L134
  constraint vertical L135
  constraint horizontal L136
  constraint vertical L137
  constraint horizontal L138
  constraint vertical L139
  constraint horizontal L140
  constraint vertical L141
  constraint horizontal L142
  constraint vertical L143
  constraint horizontal L144
  constraint vertical L145
  constraint horizontal L146
  constraint vertical L147
  constraint horizontal L148
  constraint vertical L149
  constraint horizontal L150
  constraint vertical L151
  constraint horizontal L152
  constraint vertical L153
  constraint horizontal L154
  constraint vertical L155
  constraint horizontal L156
  constraint vertical L157
  constraint horizontal L158
  constraint vertical L159
  constraint tangent L0 A0
  constraint tangent L2 A0
  constraint tangent L1 A0
  constraint tangent L3 A0
  constraint tangent L7 A1
  constraint tangent L5 A1
  constraint tangent L6 A1
  constraint tangent L4 A1
  constraint tangent L9 A2
  constraint tangent L11 A2
  constraint tangent L8 A2
  constraint tangent L10 A2
  constraint tangent L13 A3
  constraint tangent L15 A3
  constraint tangent L12 A3
  constraint tangent L14 A3
  constraint tangent L19 A4
  constraint tangent L17 A4
  constraint tangent L16 A4
  constraint tangent L18 A4
  constraint tangent L23 A5
  constraint tangent L21 A5
  constraint tangent L20 A5
  constraint tangent L22 A5
  constraint tangent L27 A6
  constraint tangent L25 A6
  constraint tangent L24 A6
  constraint tangent L26 A6
  constraint tangent L31 A7
  constraint tangent L29 A7
  constraint tangent L28 A7
  constraint tangent L30 A7
  constraint tangent L35 A8
  constraint tangent L33 A8
  constraint tangent L32 A8
  constraint tangent L34 A8
  constraint tangent L39 A9
  constraint tangent L37 A9
  constraint tangent L36 A9
  constraint tangent L38 A9
  constraint tangent L43 A10
  constraint tangent L41 A10
  constraint tangent L40 A10
  constraint tangent L42 A10
  constraint tangent L47 A11
  constraint tangent L45 A11
  constraint tangent L44 A11
  constraint tangent L46 A11
  constraint tangent L51 A12
  constraint tangent L49 A12
  constraint tangent L48 A12
  constraint tangent L50 A12
  constraint tangent L55 A13
  constraint tangent L53 A13
  constraint tangent L54 A13
  constraint tangent L52 A13
  constraint tangent L59 A14
  constraint tangent L57 A14
  constraint tangent L56 A14
  constraint tangent L58 A14
  constraint tangent L63 A15
  constraint tangent L60 A15
  constraint tangent L61 A15
  constraint tangent L62 A15
  constraint tangent L67 A16
  constraint tangent L65 A16
  constraint tangent L64 A16
  constraint tangent L66 A16
  constraint tangent L71 A17
  constraint tangent L69 A17
  constraint tangent L68 A17
  constraint tangent L70 A17
  constraint tangent L75 A18
  constraint tangent L73 A18
  constraint tangent L72 A18
  constraint tangent L74 A18
  constraint tangent L79 A19
  constraint tangent L77 A19
  constraint tangent L76 A19
  constraint tangent L78 A19
  constraint tangent L119 A20
  constraint tangent L117 A20
  constraint tangent L116 A20
  constraint tangent L118 A20
  constraint tangent L115 A21
  constraint tangent L113 A21
  constraint tangent L112 A21
  constraint tangent L114 A21
  constraint tangent L111 A22
  constraint tangent L109 A22
  constraint tangent L108 A22
  constraint tangent L110 A22
  constraint tangent L103 A23
  constraint tangent L101 A23
  constraint tangent L100 A23
  constraint tangent L102 A23
  constraint tangent L105 A24
  constraint tangent L107 A24
  constraint tangent L104 A24
  constraint tangent L106 A24
  constraint tangent L99 A25
  constraint tangent L97 A25
  constraint tangent L96 A25
  constraint tangent L98 A25
  constraint tangent L95 A26
  constraint tangent L93 A26
  constraint tangent L92 A26
  constraint tangent L94 A26
  constraint tangent L91 A27
  constraint tangent L89 A27
  constraint tangent L88 A27
  constraint tangent L90 A27
  constraint tangent L87 A28
  constraint tangent L85 A28
  constraint tangent L84 A28
  constraint tangent L86 A28
  constraint tangent L81 A29
  constraint tangent L83 A29
  constraint tangent L82 A29
  constraint tangent L80 A29
  constraint tangent L121 A30
  constraint tangent L123 A30
  constraint tangent L120 A30
  constraint tangent L122 A30
  constraint tangent L127 A31
  constraint tangent L125 A31
  constraint tangent L124 A31
  constraint tangent L126 A31
  constraint tangent L131 A32
  constraint tangent L129 A32
  constraint tangent L128 A32
  constraint tangent L130 A32
  constraint tangent L133 A33
  constraint tangent L135 A33
  constraint tangent L132 A33
  constraint tangent L134 A33
  constraint tangent L139 A34
  constraint tangent L137 A34
  constraint tangent L136 A34
  constraint tangent L138 A34
  constraint tangent L143 A35
  constraint tangent L141 A35
  constraint tangent L140 A35
  constraint tangent L142 A35
  constraint tangent L147 A36
  constraint tangent L145 A36
  constraint tangent L144 A36
  constraint tangent L146 A36
  constraint tangent L151 A37
  constraint tangent L148 A37
  constraint tangent L149 A37
  constraint tangent L150 A37
  constraint tangent L155 A38
  constraint tangent L153 A38
  constraint tangent L152 A38
  constraint tangent L154 A38
  constraint tangent L159 A39
  constraint tangent L157 A39
  constraint tangent L156 A39
  constraint tangent L158 A39
  constraint coincident L3 L160.start
  constraint coincident L0 L160.end
  constraint midpoint L160 L161.start
  constraint coincident L79 L162.start
  constraint coincident L76 L162.end
  constraint coincident L76 L163.end
  constraint midpoint L162 L164.end
  constraint equal L161 L164
  constraint coincident L119 L165.start
  constraint coincident L116 L165.end
  constraint midpoint L165 L166.end
  constraint equal L161 L166
  constraint coincident L159 L167.start
  constraint coincident L156 L167.end
  constraint midpoint L167 L168.end
  constraint equal L161 L168
  constraint tangent L160 A40
  constraint tangent L165 A41
  constraint tangent L162 A42
  constraint tangent L167 A43
  constraint coincident L161 A40.centre
  constraint equal A40 A41
  constraint coincident L166 A41.centre
  constraint equal A40 A42
  constraint coincident L164 A42.centre
  constraint coincident L168 A43.centre
  constraint equal A40 A43
  constraint coincident L47 L169.start
  constraint coincident L44 L169.end
  constraint coincident L55 L170.start
  constraint coincident L52 L170.end
  constraint coincident L63 L171.start
  constraint coincident L60 L171.end
  constraint coincident L71 L172.start
  constraint coincident L68 L172.end
  constraint coincident L111 L173.start
  constraint coincident L108 L173.end
  constraint coincident L7 L174.start
  constraint coincident L4 L174.end
  constraint coincident L11 L175.start
  constraint coincident L8 L175.end
  constraint coincident L15 L176.start
  constraint coincident L12 L176.end
  constraint coincident L19 L177.start
  constraint coincident L16 L177.end
  constraint coincident L23 L178.start
  constraint coincident L20 L178.end
  constraint coincident L27 L179.start
  constraint coincident L24 L179.end
  constraint coincident L31 L180.start
  constraint coincident L28 L180.end
  constraint coincident L35 L181.start
  constraint coincident L32 L181.end
  constraint coincident L39 L182.start
  constraint coincident L36 L182.end
  constraint midpoint L174 L183.end
  constraint midpoint L175 L184.end
  constraint perpendicular L175 L184
  constraint midpoint L176 L185.end
  constraint midpoint L177 L186.end
  constraint midpoint L178 L187.end
  constraint midpoint L179 L188.end
  constraint midpoint L180 L189.end
  constraint midpoint L181 L190.end
  constraint midpoint L182 L191.end
  constraint equal L161 L183
  constraint equal L161 L184
  constraint coincident L8.start L11.end
  constraint equal L161 L185
  constraint equal L161 L186
  constraint equal L161 L187
  constraint equal L161 L188
  constraint equal L161 L189
  constraint equal L161 L190
  constraint equal L161 L191
  constraint coincident L191 A52.centre
  constraint tangent L182 A52
  constraint tangent L181 A51
  constraint coincident L190 A51.centre
  constraint coincident L189 A50.centre
  constraint tangent L180 A50
  constraint tangent L179 A49
  constraint coincident L188 A49.centre
  constraint coincident L187 A48.centre
  constraint tangent L178 A48
  constraint tangent L177 A47
  constraint coincident L186 A47.centre
  constraint coincident L185 A46.centre
  constraint tangent L176 A46
  constraint tangent L175 A45
  constraint coincident L184 A45.centre
  constraint coincident L183 A44.centre
  constraint tangent L174 A44
  constraint equal A40 A44
  constraint equal A40 A45
  constraint equal A40 A46
  constraint equal A40 A47
  constraint equal A40 A48
  constraint equal A40 A49
  constraint equal A40 A50
  constraint equal A40 A51
  constraint equal A40 A52
  constraint coincident L43 L192.start
  constraint coincident L40 L192.end
  constraint coincident L51 L193.start
  constraint coincident L48 L193.end
  constraint coincident L59 L194.start
  constraint coincident L56 L194.end
  constraint coincident L67 L195.start
  constraint coincident L64 L195.end
  constraint coincident L75 L196.start
  constraint coincident L72 L196.end
  constraint midpoint L192 L197.end
  constraint midpoint L169 L198.end
  constraint midpoint L193 L199.end
  constraint midpoint L170 L200.end
  constraint midpoint L194 L201.end
  constraint midpoint L171 L202.end
  constraint midpoint L195 L203.end
  constraint midpoint L172 L204.end
  constraint midpoint L196 L205.end
  constraint equal L164 L205
  constraint equal L164 L204
  constraint equal L164 L203
  constraint equal L164 L202
  constraint equal L164 L201
  constraint equal L164 L200
  constraint equal L164 L199
  constraint equal L164 L198
  constraint equal L164 L197
  constraint tangent L196 A61
  constraint coincident L205 A61.centre
  constraint coincident L204 A60.centre
  constraint tangent L172 A60
  constraint tangent L195 A59
  constraint coincident L203 A59.centre
  constraint coincident L202 A58.centre
  constraint tangent L171 A58
  constraint tangent L194 A57
  constraint coincident L201 A57.centre
  constraint coincident L200 A56.centre
  constraint tangent L170 A56
  constraint tangent L193 A55
  constraint coincident L199 A55.centre
  constraint coincident L198 A54.centre
  constraint tangent L169 A54
  constraint tangent L192 A53
  constraint coincident L197 A53.centre
  constraint equal A42 A61
  constraint equal A42 A60
  constraint equal A42 A59
  constraint equal A42 A58
  constraint equal A42 A57
  constraint equal A42 A56
  constraint equal A42 A55
  constraint equal A42 A54
  constraint equal A42 A53
  constraint coincident L115 L206.start
  constraint coincident L112 L206.end
  constraint coincident L107 L207.start
  constraint coincident L104 L207.end
  constraint coincident L103 L208.start
  constraint coincident L100 L208.end
  constraint coincident L99 L209.start
  constraint coincident L96 L209.end
  constraint coincident L95 L210.start
  constraint coincident L92 L210.end
  constraint coincident L91 L211.start
  constraint coincident L88 L211.end
  constraint coincident L87 L212.start
  constraint coincident L84 L212.end
  constraint coincident L83 L213.start
  constraint coincident L80 L213.end
  constraint midpoint L212 L214.end
  constraint coincident L91 L88.start
  constraint midpoint L211 L215.end
  constraint perpendicular L211 L215
  constraint midpoint L210 L216.end
  constraint midpoint L209 L217.end
  constraint midpoint L208 L218.end
  constraint midpoint L207 L219.end
  constraint midpoint L173 L220.end
  constraint midpoint L206 L221.end
  constraint equal L166 L221
  constraint equal L166 L220
  constraint equal L166 L219
  constraint equal L166 L218
  constraint equal L166 L216
  constraint equal L166 L217
  constraint equal L166 L215
  constraint equal L166 L214
  constraint midpoint L213 L222.end
  constraint equal L166 L222
  constraint coincident L222 A69.centre
  constraint tangent L213 A69
  constraint tangent L212 A70
  constraint coincident L214 A70.centre
  constraint coincident L215 A67.centre
  constraint tangent L211 A67
  constraint tangent L210 A68
  constraint coincident L216 A68.centre
  constraint coincident L217 A65.centre
  constraint tangent L209 A65
  constraint tangent L208 A66
  constraint coincident L218 A66.centre
  constraint coincident L219 A63.centre
  constraint tangent L207 A63
  constraint tangent L173 A64
  constraint coincident L220 A64.centre
  constraint coincident L221 A62.centre
  constraint tangent L206 A62
  constraint equal A41 A62
  constraint equal A41 A64
  constraint equal A41 A63
  constraint equal A62 A66
  constraint equal A62 A65
  constraint equal A62 A68
  constraint equal A41 A67
  constraint equal A41 A70
  constraint coincident L155 L223.start
  constraint coincident L152 L223.end
  constraint coincident L151 L224.start
  constraint coincident L148 L224.end
  constraint coincident L147 L225.start
  constraint coincident L144 L225.end
  constraint coincident L143 L226.start
  constraint coincident L140 L226.end
  constraint coincident L139 L227.start
  constraint coincident L136 L227.end
  constraint coincident L135 L228.start
  constraint coincident L132 L228.end
  constraint coincident L131 L229.start
  constraint coincident L128 L229.end
  constraint coincident L127 L230.start
  constraint coincident L124 L230.end
  constraint coincident L123 L231.start
  constraint coincident L120 L231.end
  constraint midpoint L223 L232.end
  constraint midpoint L224 L233.end
  constraint midpoint L225 L234.end
  constraint midpoint L226 L235.end
  constraint midpoint L227 L236.end
  constraint midpoint L228 L237.end
  constraint midpoint L229 L238.end
  constraint midpoint L230 L239.end
  constraint midpoint L231 L240.end
  constraint equal L168 L232
  constraint equal L168 L233
  constraint equal L168 L234
  constraint equal L168 L235
  constraint equal L168 L236
  constraint equal L168 L237
  constraint equal L168 L238
  constraint equal L168 L239
  constraint equal L168 L240
  constraint tangent L231 A79
  constraint coincident L240 A79.centre
  constraint coincident L239 A78.centre
  constraint tangent L230 A78
  constraint tangent L229 A77
  constraint coincident L238 A77.centre
  constraint coincident L237 A76.centre
  constraint tangent L228 A76
  constraint tangent L227 A75
  constraint coincident L236 A75.centre
  constraint coincident L235 A74.centre
  constraint tangent L226 A74
  constraint tangent L225 A73
  constraint coincident L234 A73.centre
  constraint coincident L233 A72.centre
  constraint tangent L224 A72
  constraint tangent L223 A71
  constraint coincident L232 A71.centre
  constraint equal A43 A71
  constraint equal A43 A72
  constraint equal A43 A73
  constraint equal A43 A75
  constraint equal A43 A74
  constraint equal A43 A76
  constraint equal A43 A77
  constraint equal A43 A78
  constraint equal A43 A79
  constraint equal A41 A69
  measures "d51" angle of L0 L160
  measures "d52" distance of L0.start L161.start
  measures "d53" angle of L76 L162
  measures "d55" angle of L116 L165
  measures "d56" angle of L156 L167
  measures "d61" diameter of A40
  measures "d63" angle of L44 L169
  measures "d64" angle of L52 L170
  measures "d65" angle of L60 L171
  measures "d66" angle of L68 L172
  measures "d67" angle of L108 L173
  measures "d68" angle of L4 L174
  measures "d69" angle of L8 L175
  measures "d70" angle of L12 L176
  measures "d72" angle of L16 L177
  measures "d74" angle of L36 L182
  measures "d75" angle of L32 L181
  measures "d76" angle of L28 L180
  measures "d77" angle of L24 L179
  measures "d78" angle of L20 L178
  measures "d80" angle of L40 L192
  measures "d81" angle of L48 L193
  measures "d82" angle of L56 L194
  measures "d83" angle of L64 L195
  measures "d84" angle of L72 L196
  measures "d85" angle of L112 L206
  measures "d86" angle of L104 L207
  measures "d87" angle of L100 L208
  measures "d88" angle of L96 L209
  measures "d89" angle of L92 L210
  measures "d91" angle of L88 L211
  measures "d92" angle of L84 L212
  measures "d93" angle of L80 L213
  measures "d94" angle of L120 L231
  measures "d95" angle of L124 L230
  measures "d96" angle of L128 L229
  measures "d97" angle of L132 L228
  measures "d98" angle of L136 L227
  measures "d99" angle of L140 L226
  measures "d100" angle of L144 L225
  measures "d101" angle of L148 L224
  measures "d102" angle of L152 L223